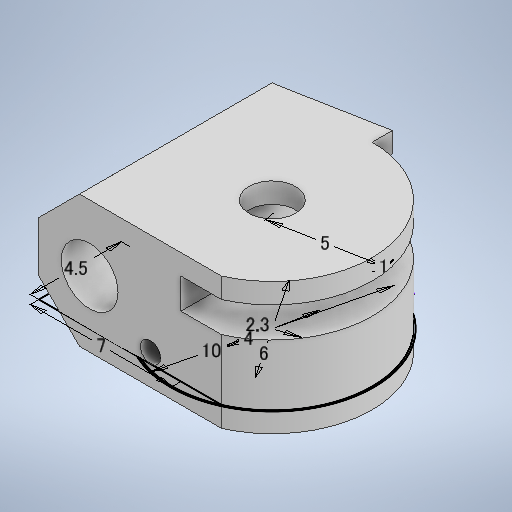
# Autodesk Inventor part: rod5.5
Saved by Autodesk Inventor 2025 (Build 290162000, 162)
## iProperties
Created: 2024-07-15
Part Number: rod5.5
Material: 一般
Document SubType Name: Modeling
Designer: Saigusa
Density: 1 g/cm^3
Appearance: 既定
Author: Saigusa
Autodesk Inventor part; units mm, degrees
ref_plane "YZ Plane" through (0, 0, 0) normal (1, 0, 0) x (0, 1, 0)
ref_plane "XZ Plane" through (0, 0, 0) normal (0, 1, 0) x (-1, 0, 0)
ref_plane "XY Plane" through (0, 0, 0) normal (0, 0, 1) x (1, 0, 0)
sketch "スケッチ1" plane through (0, 0, 0) normal (0, 1, 0) x (-1, 0, 0)
  circle A0 centre (0, 0) radius 1.15
  circle A1 centre (0, 0) radius 2
  circle A2 centre (0, 0) radius 5
  line L0 (0, 0) -> (7, 0)
  line L1 (7, 0) -> (7, 4.5)
  line L2 (7, 4.5) -> (0, 4.5)
  line L3 (0, 4.5) -> (0, 0)
  line L4 (0, 0) -> (7, 0)
  line L5 (7, 0) -> (7, -5)
  line L6 (7, -5) -> (0, -5)
  line L7 (0, -5) -> (0, 0)
  line L8 (0, 4.5) -> (-2, 4.5)
  line L9 (-2, 4.5) -> (-2, 0)
  line L10 (-2, 0) -> (0, 0)
  line L11 (0, 0) -> (0, 4.5)
  circle A3 centre (0, 0) radius 3
  line L12 (-2, 0) -> (-2, -5)
  line L13 (-2, -5) -> (0, -5)
  line L14 (2, 0) -> (2, -5)
  circle A4 centre (0, 0) radius 4.9244
  line L15 (-2, 0) -> (-4.9244, 0)
  line L16 (0, -4.9244) -> (0, -5.9244)
  line L17 (0, -5.9244) -> (7, -5.9244)
  line L18 (7, -5.9244) -> (7, -5)
  line L19 (7, -5) -> (0, -5.9244)
  line L20 (0, -5.9244) -> (4.9138, -5)
  point P0 (0, 2)
  point P1 (-2, 2.2361)
  point P2 (-2, -2.2361)
  point P3 (-2, -4.5826)
  point P4 (-2, -4.5)
  point P5 (0, -4.9244)
  dimension "d2" = 10
  dimension "d0" = 2.3
  dimension "d1" = 4
  dimension "d3" = 7
  dimension "d4" = 4.5
  dimension "d5" = 6
  dimension "d22" = 1
  dimension "d34" = 5
  constraints: 42 end point, 7 perpendicular, 7 point on line, 6 parallel, 5 coincident, 5 point on circle, 4 centre point, 4 horizontal, 2 tangent, 3 other
  measures "d0" diameter of A0
  measures "d1" diameter of A1
  measures "d3" distance of L2.end L1.end
  measures "d4" distance of L1.end L0.end
  measures "d5" diameter of A3
  measures "d22" distance of L16.start L16.end
  measures "d34" distance of L16.end L20.end
extrude "押し出し1" add sketch "スケッチ1" along normal blind 4.5 contours A1 L3 A3 L0 | L0 A3 L14 | A3 L3 L2 A4 L0 | L0 A4 L14 A3 | A4 L2 A2 L0 | L0 A2 L14 A4 | L0 L5 L6 L14 A2 | A2 L2 L1 L0
extrude "押し出し2" add sketch "スケッチ1" along normal blind 3 contours A1 L9 A3 L3 | L15 A3 L9 | L12 A3 L15 | A3 L9 L8 L3 | A3 L15 A4 L9 | L12 A4 L15 A3
extrude "押し出し3" add sketch "スケッチ1" against normal blind 1 contours L0 A1 L7 A0 | A0 L3 A1 L0 | A0 L10 A1 L3 | L7 A1 L10 A0 | L14 A3 L7 A1 | A1 L3 A3 L0 | L0 A3 L14 | A1 L9 A3 L3 | L7 A3 L12 A1 | A3 L3 L2 A4 L0 | L0 A4 L14 A3 | L14 A4 L7 A3 | L15 A3 L9 | L12 A3 L15 | A3 L9 L8 L3 | L7 A4 L12 A3 | A4 L2 A2 L0 | L0 A2 L14 A4 | L14 A2 L7 A4 | A3 L15 A4 L9 | L12 A4 L15 A3 | L0 L5 L6 L14 A2 | A2 L2 L1 L0 | L14 L6 A2 | L6 L20 L16
sketch "スケッチ2" plane through (0, 4.5, 0) normal (0, 1, 0) x (1, 0, 0)
  circle A0 centre (0, 0) radius 1.15
  circle A1 centre (0, 0) radius 2
  circle A2 centre (0, 0) radius 4.9244
  line L0 (0, 0) -> (2, 0)
  line L1 (2, 0) -> (2, -4.5)
  line L2 (2, -4.5) -> (0, -4.5)
  line L3 (0, -4.5) -> (0, 0)
  line L4 (-2, 5) -> (-7, 5) projected
  line L5 (0, -4.5) -> (-7, -4.5)
  line L6 (-7, -4.5) -> (-7, 5)
  line L7 (-7, 5) -> (0, 5)
  line L8 (0, 5) -> (0, -4.5)
  line L9 (0, 0) -> (2, 0)
  line L10 (2, 0) -> (2, 5)
  line L11 (2, 5) -> (0, 5)
  line L12 (0, 5) -> (0, 0)
  line L13 (0, 5) -> (-7, 5)
  line L14 (0, 5.9244) -> (0, 5)
  line L15 (-7, 5) -> (0, 5.9244)
  line L16 (0, 5.9244) -> (-4.9138, 5)
  line L17 (-2, 5) -> (-7, 5) projected
  point P0 (0, 4.9244)
  dimension "d12" = 4
  dimension "d35" = 5
  constraints: 32 end point, 6 parallel, 4 horizontal, 3 perpendicular, 3 point on line, 2 centre point, 2 coincident, 3 other
  measures "d12" diameter of A1
  measures "d35" distance of L14.start L16.end
extrude "押し出し4" add sketch "スケッチ2" along normal blind 1 contours L0 A1 L3 A0 | A0 L8 A1 L0 | A0 L3 A1 L8 | L1 L2 L3 A1 | L10 A2 L1 | A1 L8 A2 L10 | A1 L3 L5 A2 L8 | A2 L5 L6 L4 L7 L8 | L7 L4 L16 L14
sketch "スケッチ4" plane through (0, 3, 4.5) normal (0, 0, 1) x (1, 0, 0)
  line L0 (-7, 2.5) -> (2, 2.5) projected
  line L1 (-7, 2.5) -> (-4.5, 2.5)
  line L2 (-4.5, 2.5) -> (-4.5, -0.75)
  line L3 (-4.5, -0.75) -> (-7, -0.75)
  line L4 (-7, -0.75) -> (-7, 2.5)
  circle A0 centre (-4.5, -0.75) radius 1.4
  line L5 (0, -3) -> (0, -2.5)
  line L6 (0, -2.5) -> (-1.5, -2.5)
  circle A1 centre (-1.5, -2.5) radius 0.5
  dimension "d23" = 2.5
  dimension "d24" = 3.25
  dimension "d25" = 2.8
  dimension "d26" = 0.5
  dimension "d27" = 1.5
  dimension "d28" = 1
  constraints: 12 end point, 2 centre point, 2 coincident, 2 parallel, 2 perpendicular, 1 horizontal, 1 vertical
  measures "d23" distance of L2.end L3.end
  measures "d24" distance of L1.end L2.end
  measures "d25" diameter of A0
  measures "d26" distance of L5.start L5.end
  measures "d27" distance of L5.end L6.end
  measures "d28" diameter of A1
extrude "押し出し6" cut sketch "スケッチ4" against normal blind 6 contours A0 L3 L2 | L2 L3 A0 | A1
chamfer "面取り2" distance 2 angle 45 3 edges at (-7, 5.5, -0.25) (-7, -1, -0.25) (-7, 2.25, -5)
